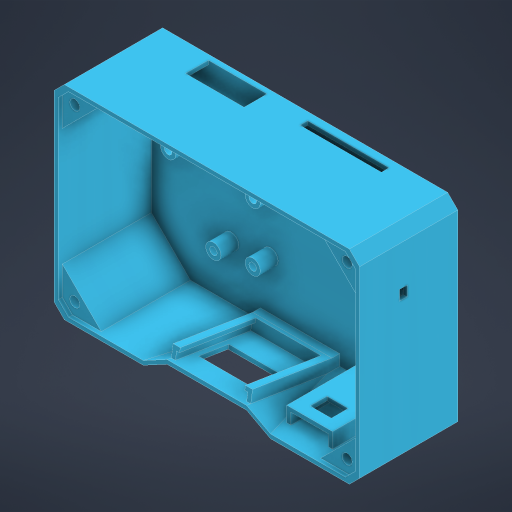
# Autodesk Inventor part: BasePlate
Saved by Autodesk Inventor 2024.2 (Build 282272000, 272)
## iProperties
Created: 2024-06-03
Part Number: BasePlate
Material: PBT Plastic
Document SubType Name: Modeling
Designer: simon
Density: 1.31 g/cm^3
Appearance: Turquoise
Author: simon
Autodesk Inventor part; units mm, degrees
ref_plane "YZ Plane" through (0, 0, 0) normal (1, 0, 0) x (0, 1, 0)
ref_plane "XZ Plane" through (0, 0, 0) normal (0, 1, 0) x (-1, 0, 0)
ref_plane "XY Plane" through (0, 0, 0) normal (0, 0, 1) x (1, 0, 0)
sketch "Sketch1" plane through (0, 0, 0) normal (0, 0, 1) x (1, 0, 0)
  line L0 (0, 0) -> (120, 0)
  line L1 (120, 0) -> (120, 80)
  line L2 (120, 80) -> (0, 80)
  line L3 (0, 80) -> (0, 0)
  dimension "d0" = 120
  dimension "d1" = 80
  constraints: 8 end point, 2 parallel, 1 horizontal, 1 perpendicular
  measures "d0" distance of L2.end L1.end
  measures "d1" distance of L1.end L0.end
extrude "Extrusion1" add sketch "Sketch1" along normal blind 2
sketch "Sketch2" plane through (0, 0, 2) normal (0, 0, 1) x (1, 0, 0)
  line L0 (0, 80) -> (0, 0) projected
  line L1 (120, 0) -> (120, 80) projected
  line L2 (0, 0) -> (120, 0)
  line L3 (120, 0) -> (120, 1.6)
  line L4 (120, 1.6) -> (0, 1.6)
  line L5 (0, 1.6) -> (0, 0)
  point P0 (0, 1.6)
  dimension "d4" = 1.6
  constraints: 8 end point, 2 parallel, 1 horizontal, 1 perpendicular, 1 point on line
  measures "d4" distance between parallel lines of L2 L4
extrude "Extrusion2" add sketch "Sketch2" along normal blind 5
ref_plane "Work Plane1" through (60, 0, 0) normal (1, 0, 0) x (0, 0, -1)
sketch "Sketch4" plane through (60, 0, 0) normal (1, 0, 0) x (0, 0, -1)
  line L0 (0, 0) -> (-7, 0) projected
  line L1 (-7, 0) -> (-38.6, 5)
  line L2 (-38.6, 5) -> (-38.6, 6.6)
  line L3 (-7, 1.6) -> (-7, 0) projected
  line L4 (-38.6, 6.6) -> (-7, 1.6)
  point P0 (-38.6, 5.8)
  dimension "d11" = 31.6
  dimension "d12" = 5
  constraints: 6 end point, 1 midpoint, 1 parallel, 1 perpendicular
  measures "d11" distance from line of point (-38.6, 5.8) L3
  measures "d12" distance from line of L1.end L0
extrude "Extrusion3" add sketch "Sketch4" along normal mid plane 31.2
sketch "Sketch5" plane through (44.4, 0, 7) normal (0, -0.9877122, 0.1562836) x (1, 0, 0)
  line L0 (3.6, 23.3931) -> (27.6, 23.3931)
  line L1 (27.6, 23.3931) -> (27.6, 11.3931)
  line L2 (27.6, 11.3931) -> (3.6, 11.3931)
  line L3 (3.6, 11.3931) -> (3.6, 23.3931)
  line L4 (0, 31.9931) -> (31.2, 31.9931) projected
  line L5 (0, 0) -> (0, 31.9931) projected
  point P0 (-44.4, -6.914)
  dimension "d15" = 24
  dimension "d16" = 12
  dimension "d17" = 8.6
  dimension "d18" = 3.6
  constraints: 8 end point, 2 parallel, 1 horizontal, 1 perpendicular
  measures "d15" distance of L1.end L2.end
  measures "d16" distance of L0.end L1.end
  measures "d17" distance between parallel lines of L4 L0
  measures "d18" distance between parallel lines of L5 L3
extrude "Extrusion4" cut sketch "Sketch5" against normal blind 2
sketch "Sketch6" plane through (44.4, 6.6, 38.6) normal (0, 0.9877122, -0.1562836) x (1, 0, 0)
  line L0 (31.2, 31.9931) -> (31.2, 0) projected
  line L1 (0, 0) -> (0, 31.9931) projected
  line L2 (31.2, 31.6441) -> (0, 31.6441)
  line L3 (0, 31.6441) -> (0, 33.2441)
  line L4 (0, 33.2441) -> (31.2, 33.2441)
  line L5 (31.2, 33.2441) -> (31.2, 31.6441)
  line L6 (3.6, 20.8501) -> (27.6, 20.8501) projected
  point P0 (-44.4, 39.1572)
  point P1 (0, 31.6441)
  dimension "d21" = 1.6
  dimension "d22" = 10.794
  constraints: 8 end point, 2 parallel, 2 point on line, 1 horizontal, 1 perpendicular
  measures "d21" distance between parallel lines of L4 L2
  measures "d22" distance between parallel lines of L6 L2
extrude "Extrusion5" add sketch "Sketch6" along normal blind 4.6
sketch "Sketch7" plane through (44.4, 1.6546, 7.3448) normal (0, 0.1562836, 0.9877122) x (1, 0, 0)
  line L0 (31.2, 0) -> (31.2, -1.5803) projected
  line L1 (0, 4.6) -> (31.2, 4.6) projected
  line L2 (31.2, 0) -> (29.6, 0)
  line L3 (29.6, 0) -> (29.6, 4.6)
  line L4 (29.6, 4.6) -> (31.2, 4.6)
  line L5 (31.2, 4.6) -> (31.2, 0)
  line L6 (0, 0) -> (-44.4, 0) projected
  line L7 (0, 0) -> (1.6, 0)
  line L8 (1.6, 0) -> (1.6, 4.6)
  line L9 (1.6, 4.6) -> (0, 4.6)
  line L10 (0, 4.6) -> (0, 0)
  line L11 (29.6, 4.6) -> (28.4, 4.6)
  line L12 (28.4, 4.6) -> (28.4, 3)
  line L13 (28.4, 3) -> (29.6, 3)
  line L14 (29.6, 3) -> (29.6, 4.6)
  line L15 (1.6, 4.6) -> (2.8, 4.6)
  line L16 (2.8, 4.6) -> (2.8, 3)
  line L17 (2.8, 3) -> (1.6, 3)
  line L18 (1.6, 3) -> (1.6, 4.6)
  point P0 (-44.4, -0.4864)
  point P1 (1.6, 3)
  point P2 (2.8, 4.6)
  dimension "d25" = 1.6
  dimension "d26" = 1.6
  dimension "d27" = 1.2
  dimension "d28" = 1.6
  dimension "d29" = 1.2
  dimension "d30" = 1.6
  constraints: 32 end point, 8 parallel, 4 horizontal, 4 perpendicular, 2 point on line
  measures "d25" distance between parallel lines of L5 L3
  measures "d26" distance between parallel lines of L10 L8
  measures "d27" distance of L13.end L12.end
  measures "d28" distance of L12.end L11.end
  measures "d29" distance of L16.end L17.end
  measures "d30" distance of L15.end L16.end
extrude "Extrusion6" add sketch "Sketch7" along normal blind 30
sketch "Sketch8" plane through (0, 0, 2) normal (0, 0, 1) x (1, 0, 0)
  line L0 (0, 1.6) -> (120, 1.6) projected
  line L1 (75.6, 1.6) -> (74, 1.6)
  line L2 (74, 1.6) -> (74, 5.93)
  line L3 (74, 5.93) -> (75.6, 5.93)
  line L4 (75.6, 5.93) -> (75.6, 1.6)
  line L5 (44.4, 1.6) -> (46, 1.6)
  line L6 (46, 1.6) -> (46, 5.93)
  line L7 (46, 5.93) -> (44.4, 5.93)
  line L8 (44.4, 5.93) -> (44.4, 1.6)
  line L9 (0, 80) -> (0, 1.6) projected
  line L10 (75.6, 5.93) -> (44.4, 5.93)
  line L11 (44.4, 5.93) -> (44.4, 4.33)
  line L12 (44.4, 4.33) -> (75.6, 4.33)
  line L13 (75.6, 4.33) -> (75.6, 5.93)
  point P0 (0, 0)
  point P1 (74.8, 5.93)
  point P2 (74, 4.33)
  point P3 (46, 4.33)
  dimension "d33" = 1.6
  dimension "d34" = 4.33
  dimension "d35" = 1.6
  dimension "d36" = 4.33
  dimension "d37" = 28
  dimension "d38" = 44.4
  dimension "d39" = 1.6
  constraints: 24 end point, 6 parallel, 3 horizontal, 3 perpendicular, 3 point on line, 1 midpoint
  measures "d33" distance of L2.end L3.end
  measures "d34" distance from line of point (74.8, 5.93) L0
  measures "d35" distance of L7.end L6.end
  measures "d36" distance of L6.end L5.end
  measures "d37" distance between parallel lines of L6 L2
  measures "d38" distance between parallel lines of L9 L8
  measures "d39" distance between parallel lines of L12 L10
extrude "Extrusion7" add sketch "Sketch8" along normal blind 4 contours L8 L12 L6 L0 | L8 L7 L6 L12 | L2 L12 L4 L0 | L6 L10 L2 L12 | L2 L3 L4 L12
sketch "Sketch10" plane through (0, 0, 7) normal (0, 0, 1) x (1, 0, 0)
  line L0 (0, 0) -> (44.4, 0) projected
  line L1 (0, 1.6) -> (120, 1.6) projected
  line L2 (0, 0) -> (35, 0)
  line L3 (35, 0) -> (35, 1.6)
  line L4 (35, 1.6) -> (0, 1.6)
  line L5 (0, 1.6) -> (0, 0)
  line L6 (120, 0) -> (120, 80) projected
  line L7 (0, 0) -> (120, 0) projected
  line L8 (120, 1.6) -> (85, 1.6)
  line L9 (85, 1.6) -> (85, 0)
  line L10 (85, 0) -> (120, 0)
  line L11 (120, 0) -> (120, 1.6)
  point P0 (44.4, 1.6)
  point P1 (0, 0.8)
  point P2 (35, 0.8)
  point P3 (120, 0.8)
  point P4 (85, 0.8)
  dimension "d42" = 35
  dimension "d43" = 35
  constraints: 16 end point, 4 midpoint, 4 parallel, 4 point on line, 2 horizontal, 2 perpendicular
  measures "d42" distance of point (0, 0.8) point (35, 0.8)
  measures "d43" distance of point (120, 0.8) point (85, 0.8)
extrude "Extrusion8" add sketch "Sketch10" along normal blind 31.6 contours L5 L1 L3 L0 | L9 L1 L6 L7
ref_plane "Work Plane8" through (35, 0, 38.6) normal (0.4650968, -0.874382, 0.1383516) x (0.2851209, 0, -0.9584916)
sketch "Sketch12" plane through (35, 0, 38.6) normal (0.4650968, -0.874382, 0.1383516) x (0.2851209, 0, -0.9584916)
  line L0 (30.2883, -7.878) -> (32.9685, 0) projected
  line L1 (30.2883, -7.878) -> (0, 0) projected
  line L2 (32.9685, 0) -> (0, 0)
  line L3 (2.6801, 10.3042) -> (11.5759, 36.4526) projected
  line L4 (0, 0) -> (2.6801, 10.3042)
  line L5 (2.6801, 10.3042) -> (32.9685, 0)
  point P0 (27.0185, -38.9562)
  constraints: 6 end point, 1 horizontal, 1 perpendicular
ref_plane "Work Plane9" through (75.6, 0, 7) normal (0.4650968, 0.874382, -0.1383516) x (0, 0.1562836, 0.9877122)
sketch "Sketch13" plane through (75.6, 0, 7) normal (0.4650968, 0.874382, -0.1383516) x (0, 0.1562836, 0.9877122)
  line L0 (31.9931, 0) -> (0, 0) projected
  line L1 (31.4618, 9.8833) -> (31.2117, 10.6184) projected
  line L2 (0, 0) -> (31.2117, 10.6184)
  line L3 (32.2432, -0.735) -> (31.9931, 0) projected
  line L4 (31.2117, 10.6184) -> (31.9931, 0)
  line L5 (31.9931, 0) -> (0, 0)
  point P0 (-6.914, -67.4345)
  constraints: 6 end point, 1 horizontal, 1 perpendicular
sketch3d "3D Sketch1"
  line L0 (44.4, 5, 38.6) -> (44.4, 6.6, 38.6)
sweep "Sweep1" add profiles "Sketch12" path "3D Sketch1" contours L2 L4 L5
sketch3d "3D Sketch2"
  line L0 (75.6, 5, 38.6) -> (75.6, 6.6, 38.6)
sweep "Sweep2" add profiles "Sketch13" path "3D Sketch2"
ref_plane "Work Plane13" through (44.4, 0, 7) normal (0, -1, 0) x (-0.2851209, 0, 0.9584916)
sketch "Sketch22" plane through (44.4, 0, 7) normal (0, -1, 0) x (-0.2851209, 0, 0.9584916)
  line L0 (0, 0) -> (-4.7925, 1.4256) projected
  line L1 (0, 0) -> (2.6801, 9.0098)
  line L2 (2.6801, 9.0098) -> (32.9685, 0)
  line L3 (32.9685, 0) -> (0, 0)
  point P0 (5.9499, 44.5529)
  point P1 (-14.3774, 4.2768)
  constraints: 6 end point, 1 horizontal, 1 perpendicular
sketch3d "3D Sketch3"
  line L0 (35, 0, 38.6) -> (35, 1.6, 38.6)
sweep "Sweep3" add profiles "Sketch22" path "3D Sketch3"
ref_plane "Work Plane14" through (75.6, 0, 7) normal (0, -1, 0) x (1, 0, 0)
sketch "Sketch23" plane through (75.6, 0, 7) normal (0, -1, 0) x (1, 0, 0)
  line L0 (0, 0) -> (9.4, 0) projected
  line L1 (9.4, 0) -> (0, 0)
  line L2 (0, 31.6) -> (9.4, 31.6) projected
  line L3 (0, 0) -> (9.4, 31.6)
  line L4 (9.4, 31.6) -> (9.4, 0)
  point P0 (-75.6, -7)
  constraints: 6 end point, 1 collinear, 1 perpendicular
sketch3d "3D Sketch4"
  line L0 (85, 0, 38.6) -> (85, 1.6, 38.6)
sweep "Sweep4" add profiles "Sketch23" path "3D Sketch4"
sketch "Sketch24" plane through (0, 0, 2) normal (0, 0, 1) x (1, 0, 0)
  line L0 (120, 80) -> (0, 80) projected
  line L1 (0, 0) -> (1.6, 0)
  line L2 (1.6, 0) -> (1.6, 80)
  line L3 (1.6, 80) -> (0, 80)
  line L4 (0, 80) -> (0, 0)
  line L5 (120, 1.6) -> (120, 80) projected
  line L6 (0, 80) -> (120, 80)
  line L7 (120, 80) -> (120, 78.4)
  line L8 (120, 78.4) -> (0, 78.4)
  line L9 (0, 78.4) -> (0, 80)
  line L10 (120, 80) -> (118.4, 80)
  line L11 (118.4, 80) -> (118.4, 0)
  line L12 (118.4, 0) -> (120, 0)
  line L13 (120, 0) -> (120, 80)
  point P0 (1.6, 78.4)
  point P1 (118.4, 78.4)
  dimension "d61" = 1.6
  dimension "d62" = 1.6
  dimension "d63" = 1.6
  constraints: 24 end point, 6 parallel, 3 horizontal, 3 perpendicular, 3 point on line
  measures "d61" distance of L3.end L2.end
  measures "d62" distance of L6.end L7.end
  measures "d63" distance of L12.end L11.end
extrude "Extrusion11" add sketch "Sketch24" along normal blind 36.6
chamfer "Chamfer1" distance 4 angle 45 8 edges at (0, 0, 19.3) (0, 80, 19.3) (120, 0, 19.3) (120, 80, 19.3) (118.4, 78.4, 20.3) (1.6, 78.4, 20.3) (118.4, 1.6, 20.3) (1.6, 1.6, 20.3)
sketch "Sketch25" plane through (4, 80, 0) normal (0, 1, 0) x (1, 0, 0)
  line L0 (110.4, -2) -> (1.6, -2) projected
  line L1 (20, -2) -> (43, -2)
  line L2 (43, -2) -> (43, -11)
  line L3 (43, -11) -> (20, -11)
  line L4 (20, -11) -> (20, -2)
  line L5 (-4, 0) -> (-4, -38.6) projected
  dimension "d69" = 23
  dimension "d70" = 9
  dimension "d71" = 24
  constraints: 8 end point, 2 parallel, 1 horizontal, 1 perpendicular, 1 point on line
  measures "d69" distance of L2.end L3.end
  measures "d70" distance of L1.end L2.end
  measures "d71" distance between parallel lines of L5 L4
extrude "Extrusion12" cut sketch "Sketch25" against normal blind 2
sketch "Sketch26" plane through (0, 0, 2) normal (0, 0, 1) x (1, 0, 0)
  line L0 (30.8, 69.4) -> (32.4, 69.4)
  line L1 (32.4, 69.4) -> (32.4, 63.4)
  line L2 (32.4, 63.4) -> (30.8, 63.4)
  line L3 (30.8, 63.4) -> (30.8, 69.4)
  line L4 (38.6, 69.4) -> (40.2, 69.4)
  line L5 (40.2, 69.4) -> (40.2, 63.4)
  line L6 (40.2, 63.4) -> (38.6, 63.4)
  line L7 (38.6, 63.4) -> (38.6, 69.4)
  line L8 (24, 80) -> (47, 80) projected
  line L9 (24, 80) -> (24, 78.4) projected
  point P0 (0, 0)
  dimension "d74" = 6
  dimension "d75" = 10.6
  dimension "d76" = 1.6
  dimension "d77" = 1.6
  dimension "d78" = 6.2
  dimension "d79" = 6.8
  constraints: 16 end point, 4 parallel, 2 horizontal, 2 perpendicular, 2 point on line
  measures "d74" distance of L2.end L0.start
  measures "d75" distance between parallel lines of L8 L0
  measures "d76" distance of L0.start L0.end
  measures "d77" distance of L4.start L4.end
  measures "d78" distance between parallel lines of L7 L1
  measures "d79" distance between parallel lines of L3 L9
extrude "Extrusion13" add sketch "Sketch26" along normal blind 9
sketch "Sketch27" plane through (4, 80, 0) normal (0, 1, 0) x (1, 0, 0)
  circle A0 centre (95.15, -9.7) radius 1.5
  circle A1 centre (57.05, -9.7) radius 1.5
  line L0 (116, -38.6) -> (116, 0) projected
  line L1 (112, 0) -> (0, 0) projected
  line L2 (60.1, -3.12) -> (92.1, -3.12)
  line L3 (92.1, -3.12) -> (92.1, -6.12)
  line L4 (92.1, -6.12) -> (60.1, -6.12)
  line L5 (60.1, -6.12) -> (60.1, -3.12)
  circle A2 centre (57.05, -9.7) radius 3
  circle A3 centre (95.15, -9.7) radius 3
  point P0 (-4, 0)
  dimension "d82" = 3
  dimension "d83" = 3
  dimension "d84" = 20.85
  dimension "d85" = 38.1
  dimension "d86" = 9.7
  dimension "d87" = 9.7
  dimension "d116" = 32
  dimension "d117" = 3
  dimension "d118" = 3.58
  dimension "d119" = 3.05
  dimension "d122" = 6
  dimension "d123" = 6
  constraints: 8 end point, 4 centre point, 2 coincident, 2 parallel, 1 horizontal, 1 perpendicular
  measures "d82" diameter of A0
  measures "d83" diameter of A1
  measures "d84" distance from line of L0 A0.centre
  measures "d85" distance of A1.centre A0.centre
  measures "d86" distance from line of A0.centre L1
  measures "d87" distance from line of A1.centre L1
  measures "d116" distance of L3.end L4.end
  measures "d117" distance of L4.end L2.start
  measures "d118" distance from line of L4 A0.centre
  measures "d119" distance from line of A0.centre L3
  measures "d122" diameter of A2
  measures "d123" diameter of A3
extrude "Extrusion14" add sketch "Sketch27" against normal blind 8.6 contours A2 | A3
sketch "Sketch28" plane through (0, 0, 2) normal (0, 0, 1) x (1, 0, 0)
  circle A0 centre (106.4, 48.4) radius 3
  circle A1 centre (106.4, 25.4) radius 3
  circle A2 centre (48.4, 48.4) radius 3
  circle A3 centre (48.4, 25.4) radius 3
  line L0 (118.4, 74.4) -> (118.4, 5.6) projected
  line L1 (5.6, 78.4) -> (114.4, 78.4) projected
  circle A4 centre (15.18, 48.4) radius 3
  circle A5 centre (32.96, 23) radius 3
  line L2 (1.6, 5.6) -> (1.6, 74.4) projected
  circle A6 centre (15.18, 48.4) radius 1.5
  circle A7 centre (48.4, 48.4) radius 1.5
  circle A8 centre (32.96, 23) radius 1.5
  circle A9 centre (106.4, 25.4) radius 1.5
  circle A10 centre (48.4, 25.4) radius 1.5
  circle A11 centre (106.4, 48.4) radius 1.5
  point P0 (0, 0)
  dimension "d90" = 6
  dimension "d91" = 6
  dimension "d92" = 6
  dimension "d93" = 6
  dimension "d94" = 23
  dimension "d95" = 23
  dimension "d96" = 58
  dimension "d97" = 12
  dimension "d98" = 30
  dimension "d101" = 6
  dimension "d102" = 6
  dimension "d103" = 30
  dimension "d104" = 13.58
  dimension "d107" = 3
  dimension "d108" = 3
  dimension "d109" = 3
  dimension "d110" = 3
  dimension "d111" = 3
  dimension "d112" = 12
  dimension "d113" = 58
  dimension "d114" = 30
  dimension "d115" = 3
  dimension "d120" = 17.78
  dimension "d121" = 25.4
  constraints: 12 centre point, 6 coincident
  measures "d90" diameter of A0
  measures "d91" diameter of A1
  measures "d92" diameter of A2
  measures "d93" diameter of A3
  measures "d94" distance of A0.centre A1.centre
  measures "d95" distance of A2.centre A3.centre
  measures "d96" distance of A1.centre A3.centre
  measures "d97" distance from line of A1.centre L0
  measures "d98" distance from line of L1 A0.centre
  measures "d101" diameter of A4
  measures "d102" diameter of A5
  measures "d103" distance from line of L1 A4.centre
  measures "d104" distance from line of L2 A4.centre
  measures "d107" diameter of A6
  measures "d108" diameter of A7
  measures "d109" diameter of A8
  measures "d110" diameter of A9
  measures "d111" diameter of A10
  measures "d112" distance from line of L0 A0.centre
  measures "d113" distance of A2.centre A0.centre
  measures "d114" distance from line of L1 A2.centre
  measures "d115" diameter of A11
  measures "d120" horizontal distance of A5.centre A4.centre
  measures "d121" vertical distance of A5.centre A4.centre
extrude "Extrusion15" add sketch "Sketch28" along normal blind 7
sketch "Sketch30" plane through (4, 80, 0) normal (0, 1, 0) x (1, 0, 0)
  line L0 (60.1, -3.12) -> (92.1, -3.12)
  line L1 (92.1, -3.12) -> (92.1, -6.12)
  line L2 (92.1, -6.12) -> (60.1, -6.12)
  line L3 (60.1, -6.12) -> (60.1, -3.12)
  circle A0 centre (95.15, -9.7) radius 3 projected
  point P0 (-4, 0)
  dimension "d130" = 32
  dimension "d131" = 3
  dimension "d136" = 3.05
  dimension "d137" = 3.58
  constraints: 8 end point, 2 parallel, 1 horizontal, 1 perpendicular
  measures "d130" distance of L1.end L3.start
  measures "d131" distance of L3.start L3.end
  measures "d136" distance from line of A0.centre L1
  measures "d137" distance from line of A0.centre L2
extrude "Extrusion16" cut sketch "Sketch30" against normal blind 2 contours L0 L1 L2 L3
sketch "Sketch31" plane through (0, 0, 2) normal (0, 0, 1) x (1, 0, 0)
  line L0 (100.15, 78.4) -> (98.15, 78.4)
  line L1 (98.15, 78.4) -> (98.15, 71.4)
  line L2 (98.15, 71.4) -> (100.15, 71.4)
  line L3 (100.15, 71.4) -> (100.15, 78.4)
  line L4 (114.4, 78.4) -> (47, 78.4) projected
  line L5 (62.05, 78.4) -> (60.05, 78.4)
  line L6 (60.05, 78.4) -> (60.05, 71.4)
  line L7 (60.05, 71.4) -> (62.05, 71.4)
  line L8 (62.05, 71.4) -> (62.05, 78.4)
  line L9 (118.4, 5.6) -> (118.4, 74.4) projected
  point P0 (0, 0)
  point P1 (99.15, 71.4)
  dimension "d140" = 2
  dimension "d141" = 2
  dimension "d142" = 7
  dimension "d143" = 36.1
  dimension "d144" = 18.25
  dimension "d146" = 7
  dimension "d147" = 7
  constraints: 16 end point, 4 parallel, 2 horizontal, 2 perpendicular, 1 midpoint, 1 point on line
  measures "d140" distance of L1.end L2.end
  measures "d141" distance of L7.end L6.end
  measures "d142" distance of L6.end L5.end
  measures "d143" distance between parallel lines of L1 L8
  measures "d144" distance between parallel lines of L3 L9
  measures "d146" distance between parallel lines of L4 L2
  measures "d147" distance from line of point (99.15, 71.4) L0
extrude "Extrusion17" add sketch "Sketch31" along normal blind 5
sketch "Sketch32" plane through (118.4, 5.6, 2) normal (-1, 0, 0) x (0, 0, 1)
  circle A0 centre (15, 52.8) radius 2.5
  circle A1 centre (15, 52.8) radius 1.5
  line L0 (0, 0) -> (0, 68.8) projected
  line L1 (23.5, 56.9) -> (17.5, 56.9)
  line L2 (17.5, 56.9) -> (17.5, 55.3)
  line L3 (17.5, 55.3) -> (23.5, 55.3)
  line L4 (23.5, 55.3) -> (23.5, 56.9)
  line L5 (23.5, 50.3) -> (17.5, 50.3)
  line L6 (17.5, 50.3) -> (17.5, 48.7)
  line L7 (17.5, 48.7) -> (23.5, 48.7)
  line L8 (23.5, 48.7) -> (23.5, 50.3)
  line L9 (15, 50.3) -> (17.5, 48.7)
  line L10 (17.9682, 50.3) -> (16.7896, 51.0543)
  line L11 (15, 55.3) -> (17.5, 56.9)
  line L12 (16.7896, 54.5457) -> (17.9682, 55.3)
  line L13 (0, 53.6) -> (12.6315, 53.6)
  line L14 (12.6315, 53.6) -> (12.6315, 52)
  line L15 (12.6315, 52) -> (0, 52)
  line L16 (0, 52) -> (0, 53.6)
  line L17 (23.5, 56.9) -> (21.9, 56.9)
  line L18 (21.9, 56.9) -> (21.9, 48.7)
  line L19 (21.9, 48.7) -> (23.5, 48.7)
  line L20 (23.5, 48.7) -> (23.5, 56.9)
  point P0 (-2, -5.6)
  point P1 (36.6, 72.8)
  point P2 (0, 52)
  point P3 (21.9, 55.3)
  point P4 (21.9, 50.3)
  dimension "d150" = 5
  dimension "d151" = 3
  dimension "d152" = 20
  dimension "d153" = 15
  dimension "d156" = 5
  dimension "d157" = 2.5
  dimension "d158" = 2.5
  dimension "d159" = 2.5
  dimension "d160" = 8.5
  dimension "d161" = 1.6
  dimension "d162" = 1.6
  dimension "d163" = 1.6
  dimension "d164" = 1.6
  dimension "d165" = 1.6
  dimension "d166" = 0.8
  dimension "d167" = 1.6
  constraints: 40 end point, 10 parallel, 5 point on circle, 5 point on line, 4 horizontal, 4 perpendicular, 2 centre point, 1 coincident
  measures "d150" diameter of A0
  measures "d151" diameter of A1
  measures "d152" vertical distance of point (36.6, 72.8) A0.centre
  measures "d153" distance from line of L0 A0.centre
  measures "d156" distance between parallel lines of L5 L3
  measures "d157" distance from line of A0.centre L3
  measures "d158" distance from line of L2 A0.centre
  measures "d159" distance from line of L6 A0.centre
  measures "d160" distance from line of L4 A0.centre
  measures "d161" distance between parallel lines of L1 L3
  measures "d162" distance between parallel lines of L7 L5
  measures "d163" distance between parallel lines of L10 L9
  measures "d164" distance between parallel lines of L12 L11
  measures "d165" distance between parallel lines of L15 L13
  measures "d166" distance from line of A0.centre L13
  measures "d167" distance between parallel lines of L20 L18
extrude "Extrusion18" add sketch "Sketch32" along normal blind 7 contours A0 L14 | A0 L11 L2 L3 L12 | L10 L5 L6 L9 A0 | L3 L2 L1 L18 | L5 L18 L7 L6 | L14 A0 | A0 L15 L0 L13 | L18 L1 L4 L3 | L3 L20 L5 L18 | L5 L8 L7 L18
sketch "Sketch33" plane through (118.4, 55.9, 23.9) normal (-1, 0, 0) x (0, 0, 1)
  line L0 (-1, 4.5) -> (-4, 4.5)
  line L1 (-4, 4.5) -> (-4, 0.5)
  line L2 (-4, 0.5) -> (-1, 0.5)
  line L3 (-1, 0.5) -> (-1, 4.5)
  line L4 (0, 5) -> (0, 0) projected
  line L5 (-3.9318, 5) -> (0, 5) projected
  point P0 (-23.9, -55.9)
  dimension "d168" = 3
  dimension "d169" = 4
  dimension "d170" = 1
  dimension "d171" = 0.5
  constraints: 8 end point, 2 parallel, 1 horizontal, 1 perpendicular
  measures "d168" distance of L2.end L1.end
  measures "d169" distance of L1.end L0.end
  measures "d170" distance between parallel lines of L4 L3
  measures "d171" distance between parallel lines of L5 L0
extrude "Extrusion19" cut sketch "Sketch33" against normal blind 2
sketch "Sketch34" plane through (0, 0, 2) normal (0, 0, 1) x (1, 0, 0)
  line L0 (102.4, 1.6) -> (100.8, 1.6)
  line L1 (100.8, 1.6) -> (100.8, 7.6)
  line L2 (100.8, 7.6) -> (102.4, 7.6)
  line L3 (102.4, 7.6) -> (102.4, 1.6)
  line L4 (102.4, 7.6) -> (86, 7.6)
  line L5 (86, 7.6) -> (86, 6)
  line L6 (86, 6) -> (102.4, 6)
  line L7 (102.4, 6) -> (102.4, 7.6)
  line L8 (86, 7.6) -> (84.4, 7.6)
  line L9 (84.4, 7.6) -> (84.4, 1.6)
  line L10 (84.4, 1.6) -> (86, 1.6)
  line L11 (86, 1.6) -> (86, 7.6)
  line L12 (75.6, 1.6) -> (114.4, 1.6) projected
  point P0 (0, 0)
  point P1 (118.4, 5.6)
  point P2 (100.8, 6)
  dimension "d174" = 1.6
  dimension "d175" = 16
  dimension "d176" = 6
  dimension "d177" = 1.6
  dimension "d179" = 1.6
  dimension "d180" = 6
  dimension "d181" = 6
  dimension "d182" = 18
  constraints: 24 end point, 6 parallel, 3 horizontal, 3 perpendicular
  measures "d174" distance between parallel lines of L4 L6
  measures "d175" distance from line of point (118.4, 5.6) L3
  measures "d176" distance between parallel lines of L12 L2
  measures "d177" distance between parallel lines of L3 L1
  measures "d179" distance between parallel lines of L9 L11
  measures "d180" distance of L8.end L9.end
  measures "d181" distance of L2.end L0.start
  measures "d182" distance between parallel lines of L9 L3
extrude "Extrusion20" add sketch "Sketch34" along normal blind 29.6 contours L0 L1 L6 L3 | L6 L1 L2 L3 | L6 L5 L4 L1 | L10 L9 L8 L5 L11
sketch "Sketch35" plane through (84.4, 7.6, 2) normal (0, 1, 0) x (1, 0, 0)
  line L0 (13.15, -25.25) -> (4.85, -25.25)
  line L1 (4.85, -25.25) -> (4.85, -18.65)
  line L2 (4.85, -18.65) -> (13.15, -18.65)
  line L3 (13.15, -18.65) -> (13.15, -25.25)
  line L4 (18, -29.6) -> (0, -29.6) projected
  line L5 (18, 0) -> (18, -29.6) projected
  point P0 (-84.4, 2)
  dimension "d185" = 8.3
  dimension "d186" = 6.6
  dimension "d187" = 4.35
  dimension "d188" = 4.85
  constraints: 8 end point, 2 parallel, 1 horizontal, 1 perpendicular
  measures "d185" distance of L1.end L2.end
  measures "d186" distance of L0.end L1.end
  measures "d187" distance between parallel lines of L4 L0
  measures "d188" distance between parallel lines of L5 L3
extrude "Extrusion21" cut sketch "Sketch35" against normal blind 2
sketch "Sketch36" plane through (44.4, 0, 7) normal (0, -1, 0) x (1, 0, 0)
  circle A0 centre (49, 16.95) radius 2
  line L0 (75.6, -7) -> (75.6, 31.6) projected
  line L1 (40.6, 31.6) -> (71.6, 31.6) projected
  point P0 (-44.4, -7)
  dimension "d191" = 4
  dimension "d192" = 26.6
  dimension "d193" = 14.65
  constraints: 1 centre point
  measures "d191" diameter of A0
  measures "d192" distance from line of A0.centre L0
  measures "d193" distance from line of L1 A0.centre
extrude "Extrusion22" cut sketch "Sketch36" against normal blind 2
sketch "Sketch37" plane through (0, 0, 2) normal (0, 0, 1) x (1, 0, 0)
  line L0 (24, 78.4) -> (5.6, 78.4) projected
  line L1 (16.9137, 78.4) -> (5.6, 78.4)
  line L2 (5.6, 78.4) -> (1.6, 74.4) projected
  line L3 (5.6, 78.4) -> (1.6, 74.4)
  line L4 (1.6, 74.4) -> (1.6, 63.0863)
  line L5 (1.6, 74.4) -> (1.6, 5.6) projected
  line L6 (1.6, 63.0863) -> (16.9137, 78.4)
  line L7 (114.4, 78.4) -> (100.15, 78.4) projected
  line L8 (103.0863, 78.4) -> (114.4, 78.4)
  line L9 (118.4, 74.4) -> (114.4, 78.4) projected
  line L10 (114.4, 78.4) -> (118.4, 74.4)
  line L11 (118.4, 74.4) -> (118.4, 63.0863)
  line L12 (118.4, 63.0863) -> (103.0863, 78.4)
  line L13 (114.4, 1.6) -> (118.4, 5.6) projected
  line L14 (118.4, 5.6) -> (114.4, 1.6)
  line L15 (114.4, 1.6) -> (103.0863, 1.6)
  line L16 (102.4, 1.6) -> (114.4, 1.6) projected
  line L17 (103.0863, 1.6) -> (118.4, 16.9137)
  line L18 (118.4, 5.6) -> (118.4, 57.6) projected
  line L19 (118.4, 16.9137) -> (118.4, 5.6)
  line L20 (5.6, 1.6) -> (44.4, 1.6) projected
  line L21 (16.9137, 1.6) -> (5.6, 1.6)
  line L22 (5.6, 1.6) -> (1.6, 5.6)
  line L23 (1.6, 5.6) -> (1.6, 16.9137)
  line L24 (1.6, 16.9137) -> (16.9137, 1.6)
  line L25 (1.6, 5.6) -> (5.6, 1.6) projected
  circle A0 centre (113.5, 73.5) radius 2
  circle A1 centre (113.5, 6.5) radius 2
  circle A2 centre (6.5, 73.5) radius 2
  circle A3 centre (6.5, 6.5) radius 2
  line L26 (0, 76) -> (0, 4) projected
  line L27 (4, 0) -> (35, 0) projected
  line L28 (85, 0) -> (116, 0) projected
  line L29 (120, 4) -> (120, 76) projected
  line L30 (116, 80) -> (4, 80) projected
  point P0 (0, 0)
  dimension "d196" = 8
  dimension "d197" = 8
  dimension "d198" = 8
  dimension "d199" = 8
  dimension "d202" = 4
  dimension "d203" = 4
  dimension "d204" = 4
  dimension "d205" = 4
  dimension "d207" = 6.5
  dimension "d208" = 6.5
  dimension "d209" = 6.5
  dimension "d210" = 6.5
  dimension "d211" = 6.5
  dimension "d212" = 6.5
  dimension "d213" = 6.5
  dimension "d214" = 6.5
  constraints: 32 end point, 7 point on line, 5 collinear, 4 centre point, 4 parallel, 2 perpendicular
  measures "d196" distance between parallel lines of L6 L2
  measures "d197" distance between parallel lines of L9 L12
  measures "d198" distance between parallel lines of L17 L13
  measures "d199" distance between parallel lines of L24 L22
  measures "d202" diameter of A0
  measures "d203" diameter of A1
  measures "d204" diameter of A2
  measures "d205" diameter of A3
  measures "d207" distance from line of L26 A3.centre
  measures "d208" distance from line of L27 A3.centre
  measures "d209" distance from line of L28 A1.centre
  measures "d210" distance from line of L29 A1.centre
  measures "d211" distance from line of L29 A0.centre
  measures "d212" distance from line of L30 A0.centre
  measures "d213" distance from line of L30 A2.centre
  measures "d214" distance from line of L26 A2.centre
extrude "Extrusion23" add sketch "Sketch37" along normal blind 35
body "Solid1"
